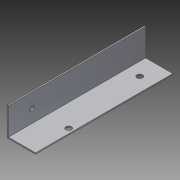
# Autodesk Inventor part: Hopper Bracing P1
Saved by Autodesk Inventor 2014 SP1 (Build 180222100, 222)
## iProperties
Created: 2013-12-15
Part Number: Hopper Bracing P1
Material: Aluminum 6061
Document SubType Name: Modeling
Designer: Moses
Mass: 7.32276 g
Surface Area: 70.4082 cm^2
Volume: 2.70213 cm^3
Density: 2.71 g/cm^3
Appearance: Aluminum - Flat
Author: Moses
Autodesk Inventor part; units mm, degrees
ref_plane "YZ Plane" through (0, 0, 0) normal (1, 0, 0) x (0, 1, 0)
ref_plane "XZ Plane" through (0, 0, 0) normal (0, 1, 0) x (-1, 0, 0)
ref_plane "XY Plane" through (0, 0, 0) normal (0, 0, 1) x (1, 0, 0)
sketch "Sketch1" plane through (0, 0, 0) normal (0, 0, 1) x (1, 0, 0)
  line L0 (0, 0) -> (0, 19.05)
  line L1 (0, 19.05) -> (0.7937, 19.05)
  line L2 (0.7937, 19.05) -> (0.7938, 0.7937)
  line L3 (0.7938, 0.7937) -> (19.05, 0.7937)
  line L4 (19.05, 0.7937) -> (19.05, 0)
  line L5 (19.05, 0) -> (0, 0)
  dimension "d0" = 19.05
  dimension "d1" = 0.7937
  constraints: 12 end point, 3 horizontal, 3 vertical, 2 perpendicular
  measures "d0" distance of L0.start L0.end
  measures "d1" distance of L0.end L1.end
extrude "Extrusion1" add sketch "Sketch1" along normal blind 92.075
sketch "Sketch2" plane through (0, 0, 0) normal (0, -1, 0) x (1, 0, 0)
  line L0 (19.05, 0) -> (0, 0) projected
  line L1 (19.05, 0) -> (19.05, 92.075) projected
  line L2 (0, 92.075) -> (19.05, 92.075) projected
  line L3 (15.875, 92.075) -> (15.875, 0) construction
  circle A0 centre (15.875, 66.675) radius 1.905
  line L4 (9.525, 92.075) -> (9.525, 0) construction
  circle A1 centre (9.525, 12.7) radius 1.905
  dimension "d4" = 3.175
  dimension "d5" = 3.81
  dimension "d6" = 25.4
  dimension "d7" = 12.7
  constraints: 4 end point, 4 point on line, 2 centre point, 2 midpoint, 1 equal radius, 1 vertical
  measures "d4" distance between parallel lines of L1 L3
  measures "d5" diameter of A0
  measures "d6" distance from line of L2 A0.centre
  measures "d7" distance from line of L0 A1.centre
extrude "Extrusion2" cut sketch "Sketch2" against normal through all
sketch "Sketch3" plane through (0, 0, 0) normal (-1, 0, 0) x (0, 0, 1)
  line L0 (0, 0) -> (0, 19.05) projected
  line L1 (92.075, 19.05) -> (92.075, 0) projected
  line L2 (0, 9.525) -> (92.075, 9.525) construction
  circle A0 centre (76.2, 9.525) radius 1.5875
  dimension "d10" = 3.175
  dimension "d11" = 15.875
  constraints: 2 end point, 2 midpoint, 1 centre point, 1 point on line
  measures "d10" diameter of A0
  measures "d11" distance from line of L1 A0.centre
extrude "Extrusion3" cut sketch "Sketch3" against normal through all
body "Solid1"
